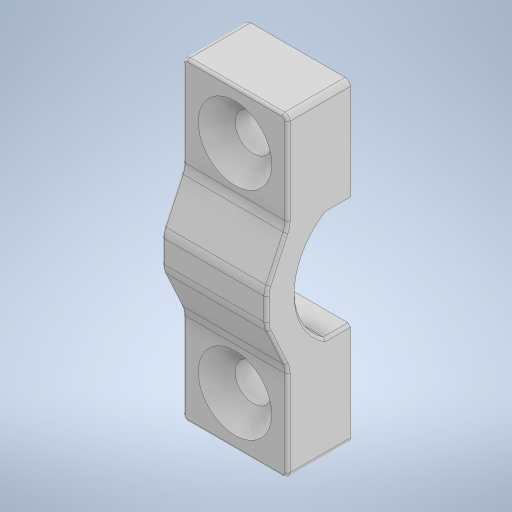
# Autodesk Inventor part: Objímka motoru pro plochu s držákem
Saved by Autodesk Inventor 2024 (Build 280153000, 153)
## iProperties
Created: 2023-08-14
Part Number: Objímka motoru pro plochu s držákem
Material: Všeobecné
Document SubType Name: Modeling
Designer: jaryj
Density: 1 g/cm^3
Appearance: Výchozí
Author: jaryj
Autodesk Inventor part; units mm, degrees
ref_plane "YZ Plane" through (0, 0, 0) normal (1, 0, 0) x (0, 1, 0)
ref_plane "XZ Plane" through (0, 0, 0) normal (0, 1, 0) x (-1, 0, 0)
ref_plane "XY Plane" through (0, 0, 0) normal (0, 0, 1) x (1, 0, 0)
sketch "Náčrt1" plane through (0, 0, 0) normal (0, 0, 1) x (1, 0, 0)
  line L0 (-5, 15) -> (5, 15)
  line L1 (5, 15) -> (5, -15)
  line L2 (5, -15) -> (-5, -15)
  line L3 (-5, -15) -> (-5, 15)
  line L4 (-5, 15) -> (5, -15) construction
  line L5 (5, 15) -> (-5, -15) construction
  circle A0 centre (0, 10.3125) radius 1.5
  circle A1 centre (0, -10.3125) radius 1.5
  line L6 (-5, 0) -> (5, 0)
  line L7 (0, 10.3125) -> (0, 15) construction
  line L8 (0, -10.3125) -> (0, -15) construction
  point P0 (0, 0)
  dimension "d0" = 30
  dimension "d1" = 10
  dimension "d2" = 3
  dimension "d42" = 20.625
  constraints: 18 end point, 6 midpoint, 2 centre point, 2 parallel, 2 vertical alignment, 1 equal radius, 1 horizontal, 1 perpendicular, 1 vertical, 1 other
  measures "d0" distance of L2.end L0.start
  measures "d1" distance of L0.start L0.end
  measures "d2" diameter of A0
  measures "d42" distance of L8.start L7.start
extrude "Vysunutí1" add sketch "Náčrt1" along normal blind 10
sketch "Náčrt2" plane through (5, -15, 0) normal (1, 0, 0) x (0, 0, -1)
  line L0 (0, 0) -> (0, 30) projected
  line L1 (0, 10) -> (-3.3166, 10)
  arc A0 (-3.3166, 20) -> (-3.3166, 10) centre (0, 15) ccw
  line L2 (-3.3166, 20) -> (0, 20)
  line L3 (0, 9.875) -> (-3.3541, 9.875)
  arc A1 (-3.3541, 20.125) -> (-3.3541, 9.875) centre (0, 15) ccw
  line L4 (-3.3541, 20.125) -> (0, 20.125)
  line L5 (0, 30) -> (-10, 30) projected
  line L6 (0, 6.875) -> (-4.1533, 6.875) construction
  arc A2 (-4.1533, 23.125) -> (-4.1533, 6.875) centre (0, 15) ccw construction
  line L7 (-4.1533, 23.125) -> (0, 23.125) construction
  line L8 (0, 0) -> (-10, 0) projected
  line L9 (-7, 0) -> (-7, 9.1463)
  line L10 (-7, 9.1463) -> (-9, 13.4948)
  line L11 (-9, 16.5052) -> (-7, 20.8537)
  line L12 (-7, 20.8537) -> (-7, 30)
  line L13 (-9, 13.4948) -> (-9, 16.5052)
  line L14 (-10, 0) -> (-10, 30) projected
  point P0 (0, 9.875)
  point P1 (-9, 15)
  point P2 (-10, 15)
  dimension "d7" = 6
  dimension "d8" = 10
  dimension "d9" = 0.125
  dimension "d16" = 3
  dimension "d17" = 3
  dimension "d18" = 3
  dimension "d19" = 1
  constraints: 22 end point, 10 point on circle, 4 midpoint, 4 parallel, 4 point on line, 3 centre point, 2 coincident, 2 vertical, 1 horizontal, 1 horizontal alignment, 1 perpendicular, 4 other
  measures "d7" radius of A0
  measures "d8" distance between parallel lines of L2 L1
  measures "d9" distance between parallel lines of L1 L3
  measures "d16" radial gap between concentric circles of A1 A2
  measures "d17" distance between parallel lines of L14 L9
  measures "d18" distance between parallel lines of L14 L12
  measures "d19" distance between parallel lines of L14 L13
extrude "Vysunutí2" cut sketch "Náčrt2" against normal through all contours L3 A1 L4 L0 L2 A0 L1 | L8 L14 L5 L12 L11 L13 L10 L9 | L1 A0 L2 L0
fillet "Zaoblení1" radius 2 4 edges at (0, -1.5052, 9) (0, 1.5052, 9) (0, 5.8537, 7) (0, -5.8537, 7)
fillet "Zaoblení2" radius 0.25 20 edges at (0, -15, 7) (0, 15, 7) (5, -5.8638, 7.0463) (5, -3.6794, 8) (5, -1.4951, 8.9537) (5, 0, 9) (5, 1.4951, 8.9537) (5, 3.6794, 8) (5, 5.8638, 7.0463) (5, 10.6458, 7) (5, -10.6458, 7) (-5, -5.8638, 7.0463) (-5, -3.6794, 8) (-5, -1.4951, 8.9537) (-5, 0, 9) (-5, 1.4951, 8.9537) (-5, 3.6794, 8) (-5, 5.8638, 7.0463) (-5, 10.6458, 7) (-5, -10.6458, 7)
sketch "Náčrt3" plane through (0, 0, 0) normal (0, 0, -1) x (-1, 0, 0)
  line L0 (5, -5.125) -> (-5, -5.125) projected
  line L1 (-5, -15) -> (-5, -5.125) projected
  line L2 (5, -15) -> (-5, -15) projected
  line L3 (5, -5.125) -> (5, -15) projected
  circle A0 centre (0, -10.3125) radius 1.5 projected
  line L4 (-5, 5.125) -> (5, 5.125) projected
  line L5 (5, 15) -> (5, 5.125) projected
  line L6 (-5, 15) -> (5, 15) projected
  line L7 (-5, 5.125) -> (-5, 15) projected
  circle A1 centre (0, 10.3125) radius 1.5 projected
  point P0 (0, 0)
extrude "Vysunutí3" cut sketch "Náčrt3" against normal blind 1
chamfer "Zkosení1" distance 0.25 angle 45 6 edges at (5, -5.125, 2.1771) (5, 0, 6.125) (5, 5.125, 2.1771) (-5, -5.125, 2.1771) (-5, 0, 6.125) (-5, 5.125, 2.1771)
fillet "Zaoblení3" radius 0.5 8 edges at (4.9268, -14.9268, 6.9268) (5, -15, 3.875) (-4.9268, -14.9268, 6.9268) (-5, -15, 3.875) (-4.9268, 14.9268, 6.9268) (-5, 15, 3.875) (4.9268, 14.9268, 6.9268) (5, 15, 3.875)
sketch "Náčrt4" plane through (-4.75, 6.2916, 7) normal (0, 0, 1) x (1, 0, 0)
  circle A0 centre (4.75, 4.0209) radius 1.5 projected
  point P0 (4.75, -6.2916)
  constraints: 1 coincident
hole "Díra1" at (0, 10.3125, 7) direction (0, 0, -1) diameter 3.5 end through all countersink diameter 7 countersink angle 90
sketch "Náčrt5" plane through (-4.75, -6.2916, 7) normal (0, 0, 1) x (1, 0, 0)
  circle A0 centre (4.75, -4.0209) radius 1.5 projected
  point P0 (4.75, 6.2916)
  constraints: 1 coincident
hole "Díra2" at (0, -10.3125, 7) direction (0, 0, -1) diameter 3.5 end through all countersink diameter 7 countersink angle 90
